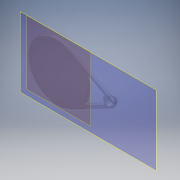
# Autodesk Inventor part: trapdoor_servo
Saved by Autodesk Inventor 2019 (Build 230136000, 136)
## iProperties
Created: 2019-01-09
Part Number: trapdoor_servo
Material: PET Plastic
Document SubType Name: Modeling
Designer: jmc
Density: 1.541 g/cm^3
Appearance: Polycarbonate - Clear
Author: jmc
Autodesk Inventor part; units mm, degrees
ref_plane "YZ Plane" through (0, 0, 0) normal (1, 0, 0) x (0, 1, 0)
ref_plane "XZ Plane" through (0, 0, 0) normal (0, 1, 0) x (-1, 0, 0)
ref_plane "XY Plane" through (0, 0, 0) normal (0, 0, 1) x (1, 0, 0)
ref_plane "Work Plane1" through (0, 0, 0) normal (0, 0, -1) x (-1, 0, 0)
ref_plane "Work Plane3" through (-59.1654, 22.8024, -1.2767) normal (0, 0, 1) x (0, 1, 0)
sketch "Sketch4" plane through (-59.1654, 22.8024, -1.2767) normal (0, 0, 1) x (0, 1, 0)
  line L0 (0, 0.2578) -> (0, -48.4285) construction
  line L1 (-4.3051, -44.7422) -> (4.9106, -44.7422) construction
  circle A0 centre (0, -44.7422) radius 2.97
  circle A1 centre (0, 0) radius 25.1499 construction
  arc A2 (-4.4358, -46.9838) -> (4.4358, -46.9838) centre (0, -44.7422) ccw
  line L2 (0, -55.7616) -> (-22.5832, -11.0728)
  line L3 (0, -55.7616) -> (22.4465, -11.3432)
  arc A3 (22.4465, -11.3432) -> (-22.4465, -11.3432) centre (0, 0) ccw
  line L4 (0, 0) -> (0, -25.1499) construction
  line L5 (0, -41.7722) -> (0, -73.1545) construction
  point P0 (-22.8024, -59.1654)
  dimension "d9" = 5.94
  dimension "d8" = 45
  dimension "d10" = 2
  constraints: 12 end point, 7 point on circle, 6 point on line, 3 centre point, 3 coincident, 3 vertical, 2 tangent, 1 concentric, 1 horizontal, 1 vertical alignment, 2 other
  measures "d8" distance from line of L0.start L1
extrude "Extrusion2" add sketch "Sketch4" along normal blind 2 contours L2 A3 L3 A2
fillet "Fillet2" radius 1.5 4 edges at (-9.4532, 22.8024, 0.7233) (-30.0019, 36.2436, 0.7233) (-84.3153, 22.8024, 0.7233) (-30.0019, 9.3612, 0.7233)
sketch "Sketch5" plane through (-59.1654, 22.8024, 0.7233) normal (0, 0, 1) x (1, 0, 0)
  line L0 (41.0298, 3.3493) -> (24.2777, 11.8149)
  line L1 (24.2777, -11.8149) -> (41.0298, -3.3493)
  line L2 (11.3432, -22.4465) -> (46.9838, -4.4358) projected
  line L3 (46.9838, 4.4358) -> (11.3432, 22.4465) projected
  arc A0 (46.9838, -4.4358) -> (46.9838, 4.4358) centre (44.7422, 0) ccw projected
  circle A1 centre (44.7422, 0) radius 2.97 projected
  arc A2 (46.3073, -3.097) -> (46.3073, 3.097) centre (44.7422, 0) ccw projected
  line L4 (10.6667, 21.1078) -> (46.3073, 3.097) projected
  arc A3 (10.6667, 21.1078) -> (10.6667, -21.1078) centre (0, 0) ccw projected
  line L5 (46.3073, -3.097) -> (10.6667, -21.1078) projected
  line L6 (-0.2578, 0) -> (48.4285, 0) construction
  arc A4 (24.2777, -11.8149) -> (24.2777, 11.8149) centre (0, 0) ccw
  arc A5 (41.0298, 3.3493) -> (41.0298, -3.3493) centre (44.7422, 0) ccw
  line L7 (48.7042, -0.0038) -> (-50.8727, 0.004) construction
  point P0 (59.1654, -22.8024)
  point P1 (39.7422, -4)
  point P2 (39.7422, 4)
  point P3 (26.5473, 10.668)
  point P4 (26.5473, -10.668)
  dimension "d25" = 27
  dimension "d27" = 5
  constraints: 4 end point, 4 point on circle, 4 point on line, 2 centre point, 2 coincident, 2 parallel, 1 other
  measures "d25" radius of A4
  measures "d27" radius of A5
extrude "Extrusion3" cut sketch "Sketch5" against normal through all contours A5 L1 A4 L0
fillet "Fillet4" radius 1 4 edges at (-18.1356, 26.1517, -0.2767) (-18.1356, 19.4531, -0.2767) (-34.8877, 34.6173, -0.2767) (-34.8877, 10.9875, -0.2767)
fillet "Fillet5" radius 1 8 edges at (-33.56, 12.3687, 0.7233) (-32.1654, 22.8024, 0.7233) (-33.56, 33.2361, 0.7233) (-25.8107, 30.0303, 0.7233) (-18.6709, 26.073, 0.7233) (-19.4232, 22.8024, 0.7233) (-18.6709, 19.5318, 0.7233) (-25.8107, 15.5745, 0.7233)
sketch "Sketch6" plane through (-59.1654, 22.8024, -1.2767) normal (0, 0, -1) x (-1, 0, 0)
  line L0 (-47.2622, 0) -> (-42.2222, 0) construction
  circle A0 centre (-44.7422, 0) radius 4.17
  arc A1 (-46.9838, 4.4358) -> (-46.9838, -4.4358) centre (-44.7422, 0) ccw construction
  point P0 (-59.1654, -22.8024)
  dimension "d30" = 0.8
  constraints: 2 end point, 1 centre point, 1 horizontal, 1 midpoint, 2 other
  measures "d30" radial gap between concentric circles of A1 A0
extrude "Extrusion4" add sketch "Sketch6" along normal blind 2.62
fillet "Fillet6" radius 1 1 edges at (-10.2532, 22.8024, -3.8967)
sketch "Sketch7" plane through (-14.4232, 22.8024, -1.2767) normal (0, 0, 1) x (1, 0, 0)
  circle A0 centre (0, 0) radius 2.97 projected
  point P0 (14.4232, -22.8024)
extrude "Extrusion5" cut sketch "Sketch7" against normal blind 1.82
sketch "Sketch8" plane through (-14.4232, 22.8024, -3.8967) normal (0, 0, -1) x (-1, 0, 0)
  circle A0 centre (0, 0) radius 1.3 projected
  point P0 (-14.4232, -22.8024)
hole "Hole1" at (-14.4232, 22.8024, -3.8967) direction (0, 0, 1) diameter 2.86 depth 1.82 countersink diameter 5.65 countersink angle 90
fillet "Fillet7" radius 0.5 1 edges at (-10.2532, 22.8024, -1.2767)
body "Solid2"
